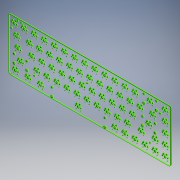
# Autodesk Inventor part: 60pc_pcb.kicad_v1.1_pcb.kicad_pcb
Saved by Autodesk Inventor 2018 (Build 220112000, 112)
## iProperties
Created: 2018-02-17
Part Number: 60pc_pcb.kicad_v1.1_pcb.kicad_pcb
Material: Generic
Document SubType Name: Modeling
Designer: ConnorDevitt
Density: 1 g/cm^3
Appearance: Board Outline
Author: ConnorDevitt
Autodesk Inventor part; units mm, degrees
(part 1 of 2)
ref_plane "YZ Plane" through (0, 0, 0) normal (1, 0, 0) x (0, 1, 0)
ref_plane "XZ Plane" through (0, 0, 0) normal (0, 1, 0) x (-1, 0, 0)
ref_plane "XY Plane" through (0, 0, 0) normal (0, 0, 1) x (1, 0, 0)
sketch "Sketch1" plane through (0, 0, 0) normal (0, 0, 1) x (1, 0, 0)
  line L0 (-153.375, 46.5) -> (-153.375, 43.75)
  line L1 (-153.375, 43.75) -> (-153.375, -45.25)
  arc A0 (-153.375, -45.25) -> (-149.375, -49.25) centre (-149.375, -45.25) ccw
  line L2 (-149.375, -49.25) -> (-147.625, -49.25)
  line L3 (-147.625, -49.25) -> (142.375, -49.25)
  line L4 (142.375, -49.25) -> (145.625, -49.25)
  line L5 (145.625, -49.25) -> (146.875, -49.25)
  line L6 (146.875, -49.25) -> (149.375, -49.25)
  arc A1 (149.375, -49.25) -> (153.375, -45.25) centre (149.375, -45.25) ccw
  line L7 (153.375, -45.25) -> (153.375, -18.5)
  line L8 (153.375, -18.5) -> (153.375, 46.5)
  arc A2 (153.375, 46.5) -> (150.625, 49.25) centre (150.625, 46.5) ccw
  line L9 (150.625, 49.25) -> (150.125, 49.25)
  line L10 (150.125, 49.25) -> (148.125, 49.25)
  line L11 (148.125, 49.25) -> (140.875, 49.25)
  line L12 (140.875, 49.25) -> (-127.875, 49.25)
  line L13 (-127.875, 49.25) -> (-128.125, 49.25)
  line L14 (-128.125, 49.25) -> (-148.875, 49.25)
  line L15 (-148.875, 49.25) -> (-150.625, 49.25)
  arc A3 (-150.625, 49.25) -> (-153.375, 46.5) centre (-150.625, 46.5) ccw
  line L16 (-126.3127, 41.7733) -> (-127.1236, 40.3134)
  arc A4 (-128.4349, 41.0417) -> (-127.1236, 40.3134) centre (-127.7792, 40.6775) ccw
  line L17 (-128.4349, 41.0417) -> (-127.6239, 42.5016)
  arc A5 (-126.3127, 41.7733) -> (-127.6239, 42.5016) centre (-126.9683, 42.1375) ccw
  line L18 (-120.6808, 43.1658) -> (-120.7202, 42.5872)
  arc A6 (-122.2167, 42.6892) -> (-120.7202, 42.5872) centre (-121.4685, 42.6382) ccw
  line L19 (-122.2167, 42.6892) -> (-122.1773, 43.2678)
  arc A7 (-120.6808, 43.1658) -> (-122.1773, 43.2678) centre (-121.429, 43.2168) ccw
  line L20 (-145.3627, 41.7733) -> (-146.1736, 40.3134)
  arc A8 (-147.4848, 41.0417) -> (-146.1736, 40.3134) centre (-146.8292, 40.6775) ccw
  line L21 (-147.4848, 41.0417) -> (-146.6739, 42.5016)
  arc A9 (-145.3627, 41.7733) -> (-146.6739, 42.5016) centre (-146.0183, 42.1375) ccw
  line L22 (-139.7308, 43.1658) -> (-139.7702, 42.5872)
  arc A10 (-141.2667, 42.6892) -> (-139.7702, 42.5872) centre (-140.5185, 42.6382) ccw
  line L23 (-141.2667, 42.6892) -> (-141.2273, 43.2678)
  arc A11 (-139.7308, 43.1658) -> (-141.2273, 43.2678) centre (-140.479, 43.2168) ccw
  line L24 (-136.925, 46.4) -> (-136.925, 43.9)
  arc A12 (-137.625, 43.9) -> (-136.925, 43.9) centre (-137.275, 43.9) ccw
  line L25 (-137.625, 43.9) -> (-137.625, 46.4)
  arc A13 (-136.925, 46.4) -> (-137.625, 46.4) centre (-137.275, 46.4) ccw
  line L26 (-129.625, 46.4) -> (-129.625, 43.9)
  arc A14 (-130.325, 43.9) -> (-129.625, 43.9) centre (-129.975, 43.9) ccw
  line L27 (-130.325, 43.9) -> (-130.325, 46.4)
  arc A15 (-129.625, 46.4) -> (-130.325, 46.4) centre (-129.975, 46.4) ccw
  line L28 (-140.6002, 22.7233) -> (-141.4111, 21.2634)
  arc A16 (-142.7224, 21.9917) -> (-141.4111, 21.2634) centre (-142.0667, 21.6275) ccw
  line L29 (-142.7224, 21.9917) -> (-141.9114, 23.4516)
  arc A17 (-140.6002, 22.7233) -> (-141.9114, 23.4516) centre (-141.2558, 23.0875) ccw
  line L30 (-134.9683, 24.1158) -> (-135.0077, 23.5372)
  arc A18 (-136.5042, 23.6392) -> (-135.0077, 23.5372) centre (-135.756, 23.5882) ccw
  line L31 (-136.5042, 23.6392) -> (-136.4648, 24.2178)
  arc A19 (-134.9683, 24.1158) -> (-136.4648, 24.2178) centre (-135.7165, 24.1668) ccw
  line L32 (-138.2189, 3.6733) -> (-139.0298, 2.2134)
  arc A20 (-140.3411, 2.9417) -> (-139.0298, 2.2134) centre (-139.6855, 2.5775) ccw
  line L33 (-140.3411, 2.9417) -> (-139.5302, 4.4016)
  arc A21 (-138.2189, 3.6733) -> (-139.5302, 4.4016) centre (-138.8745, 4.0375) ccw
  line L34 (-132.587, 5.0658) -> (-132.6265, 4.4872)
  arc A22 (-134.123, 4.5892) -> (-132.6265, 4.4872) centre (-133.3747, 4.5382) ccw
  line L35 (-134.123, 4.5892) -> (-134.0835, 5.1678)
  arc A23 (-132.587, 5.0658) -> (-134.0835, 5.1678) centre (-133.3353, 5.1168) ccw
  line L36 (-133.4564, -15.3767) -> (-134.2673, -16.8366)
  arc A24 (-135.5786, -16.1083) -> (-134.2673, -16.8366) centre (-134.923, -16.4725) ccw
  line L37 (-135.5786, -16.1083) -> (-134.7677, -14.6484)
  arc A25 (-133.4564, -15.3767) -> (-134.7677, -14.6484) centre (-134.112, -15.0125) ccw
  line L38 (-127.8245, -13.9842) -> (-127.864, -14.5628)
  arc A26 (-129.3605, -14.4608) -> (-127.864, -14.5628) centre (-128.6122, -14.5118) ccw
  line L39 (-129.3605, -14.4608) -> (-129.321, -13.8822)
  arc A27 (-127.8245, -13.9842) -> (-129.321, -13.8822) centre (-128.5728, -13.9332) ccw
  line L40 (-142.9814, -34.4267) -> (-143.7923, -35.8866)
  arc A28 (-145.1036, -35.1583) -> (-143.7923, -35.8866) centre (-144.448, -35.5225) ccw
  line L41 (-145.1036, -35.1583) -> (-144.2927, -33.6984)
  arc A29 (-142.9814, -34.4267) -> (-144.2927, -33.6984) centre (-143.637, -34.0625) ccw
  line L42 (-137.3495, -33.0342) -> (-137.389, -33.6128)
  arc A30 (-138.8855, -33.5108) -> (-137.389, -33.6128) centre (-138.1372, -33.5618) ccw
  line L43 (-138.8855, -33.5108) -> (-138.846, -32.9322)
  arc A31 (-137.3495, -33.0342) -> (-138.846, -32.9322) centre (-138.0978, -32.9832) ccw
  line L44 (-116.7876, 22.7233) -> (-117.5986, 21.2634)
  arc A32 (-118.9099, 21.9917) -> (-117.5986, 21.2634) centre (-118.2542, 21.6275) ccw
  line L45 (-118.9099, 21.9917) -> (-118.0989, 23.4516)
  arc A33 (-116.7876, 22.7233) -> (-118.0989, 23.4516) centre (-117.4433, 23.0875) ccw
  line L46 (-111.1558, 24.1158) -> (-111.1952, 23.5372)
  arc A34 (-112.6917, 23.6392) -> (-111.1952, 23.5372) centre (-111.9435, 23.5882) ccw
  line L47 (-112.6917, 23.6392) -> (-112.6523, 24.2178)
  arc A35 (-111.1558, 24.1158) -> (-112.6523, 24.2178) centre (-111.904, 24.1668) ccw
  line L48 (-112.0251, 3.6733) -> (-112.8361, 2.2134)
  arc A36 (-114.1474, 2.9417) -> (-112.8361, 2.2134) centre (-113.4917, 2.5775) ccw
  line L49 (-114.1474, 2.9417) -> (-113.3364, 4.4016)
  arc A37 (-112.0251, 3.6733) -> (-113.3364, 4.4016) centre (-112.6808, 4.0375) ccw
  line L50 (-106.3933, 5.0658) -> (-106.4327, 4.4872)
  arc A38 (-107.9292, 4.5892) -> (-106.4327, 4.4872) centre (-107.181, 4.5382) ccw
  line L51 (-107.9292, 4.5892) -> (-107.8898, 5.1678)
  arc A39 (-106.3933, 5.0658) -> (-107.8898, 5.1678) centre (-107.1415, 5.1168) ccw
  line L52 (-102.5002, -15.3767) -> (-103.3111, -16.8366)
  arc A40 (-104.6223, -16.1083) -> (-103.3111, -16.8366) centre (-103.9667, -16.4725) ccw
  line L53 (-104.6223, -16.1083) -> (-103.8114, -14.6484)
  arc A41 (-102.5002, -15.3767) -> (-103.8114, -14.6484) centre (-103.1558, -15.0125) ccw
  line L54 (-96.8683, -13.9842) -> (-96.9077, -14.5628)
  arc A42 (-98.4042, -14.4608) -> (-96.9077, -14.5628) centre (-97.656, -14.5118) ccw
  line L55 (-98.4042, -14.4608) -> (-98.3648, -13.8822)
  arc A43 (-96.8683, -13.9842) -> (-98.3648, -13.8822) centre (-97.6165, -13.9332) ccw
  line L56 (-119.1689, -34.4267) -> (-119.9798, -35.8866)
  arc A44 (-121.2911, -35.1583) -> (-119.9798, -35.8866) centre (-120.6355, -35.5225) ccw
  line L57 (-121.2911, -35.1583) -> (-120.4802, -33.6984)
  arc A45 (-119.1689, -34.4267) -> (-120.4802, -33.6984) centre (-119.8245, -34.0625) ccw
  line L58 (-113.537, -33.0342) -> (-113.5765, -33.6128)
  arc A46 (-115.073, -33.5108) -> (-113.5765, -33.6128) centre (-114.3247, -33.5618) ccw
  line L59 (-115.073, -33.5108) -> (-115.0335, -32.9322)
  arc A47 (-113.537, -33.0342) -> (-115.0335, -32.9322) centre (-114.2853, -32.9832) ccw
  line L60 (-95.3564, -34.4267) -> (-96.1673, -35.8866)
  arc A48 (-97.4786, -35.1583) -> (-96.1673, -35.8866) centre (-96.823, -35.5225) ccw
  line L61 (-97.4786, -35.1583) -> (-96.6677, -33.6984)
  arc A49 (-95.3564, -34.4267) -> (-96.6677, -33.6984) centre (-96.012, -34.0625) ccw
  line L62 (-89.7245, -33.0342) -> (-89.764, -33.6128)
  arc A50 (-91.2605, -33.5108) -> (-89.764, -33.6128) centre (-90.5122, -33.5618) ccw
  line L63 (-91.2605, -33.5108) -> (-91.221, -32.9322)
  arc A51 (-89.7245, -33.0342) -> (-91.221, -32.9322) centre (-90.4728, -32.9832) ccw
  line L64 (-107.2626, 41.7733) -> (-108.0736, 40.3134)
  arc A52 (-109.3849, 41.0417) -> (-108.0736, 40.3134) centre (-108.7292, 40.6775) ccw
  line L65 (-109.3849, 41.0417) -> (-108.5739, 42.5016)
  arc A53 (-107.2626, 41.7733) -> (-108.5739, 42.5016) centre (-107.9183, 42.1375) ccw
  line L66 (-101.6308, 43.1658) -> (-101.6702, 42.5872)
  arc A54 (-103.1667, 42.6892) -> (-101.6702, 42.5872) centre (-102.4185, 42.6382) ccw
  line L67 (-103.1667, 42.6892) -> (-103.1273, 43.2678)
  arc A55 (-101.6308, 43.1658) -> (-103.1273, 43.2678) centre (-102.379, 43.2168) ccw
  line L68 (-97.7377, 22.7233) -> (-98.5486, 21.2634)
  arc A56 (-99.8598, 21.9917) -> (-98.5486, 21.2634) centre (-99.2042, 21.6275) ccw
  line L69 (-99.8598, 21.9917) -> (-99.0489, 23.4516)
  arc A57 (-97.7377, 22.7233) -> (-99.0489, 23.4516) centre (-98.3933, 23.0875) ccw
  line L70 (-92.1058, 24.1158) -> (-92.1452, 23.5372)
  arc A58 (-93.6417, 23.6392) -> (-92.1452, 23.5372) centre (-92.8935, 23.5882) ccw
  line L71 (-93.6417, 23.6392) -> (-93.6023, 24.2178)
  arc A59 (-92.1058, 24.1158) -> (-93.6023, 24.2178) centre (-92.854, 24.1668) ccw
  line L72 (-92.9752, 3.6733) -> (-93.7861, 2.2134)
  arc A60 (-95.0974, 2.9417) -> (-93.7861, 2.2134) centre (-94.4417, 2.5775) ccw
  line L73 (-95.0974, 2.9417) -> (-94.2864, 4.4016)
  arc A61 (-92.9752, 3.6733) -> (-94.2864, 4.4016) centre (-93.6308, 4.0375) ccw
  line L74 (-87.3433, 5.0658) -> (-87.3827, 4.4872)
  arc A62 (-88.8792, 4.5892) -> (-87.3827, 4.4872) centre (-88.131, 4.5382) ccw
  line L75 (-88.8792, 4.5892) -> (-88.8398, 5.1678)
  arc A63 (-87.3433, 5.0658) -> (-88.8398, 5.1678) centre (-88.0915, 5.1168) ccw
  line L76 (-83.4502, -15.3767) -> (-84.2611, -16.8366)
  arc A64 (-85.5724, -16.1083) -> (-84.2611, -16.8366) centre (-84.9167, -16.4725) ccw
  line L77 (-85.5724, -16.1083) -> (-84.7614, -14.6484)
  arc A65 (-83.4502, -15.3767) -> (-84.7614, -14.6484) centre (-84.1058, -15.0125) ccw
  line L78 (-77.8183, -13.9842) -> (-77.8577, -14.5628)
  arc A66 (-79.3542, -14.4608) -> (-77.8577, -14.5628) centre (-78.606, -14.5118) ccw
  line L79 (-79.3542, -14.4608) -> (-79.3148, -13.8822)
  arc A67 (-77.8183, -13.9842) -> (-79.3148, -13.8822) centre (-78.5665, -13.9332) ccw
  line L80 (-88.2126, 41.7733) -> (-89.0236, 40.3134)
  arc A68 (-90.3349, 41.0417) -> (-89.0236, 40.3134) centre (-89.6792, 40.6775) ccw
  line L81 (-90.3349, 41.0417) -> (-89.5239, 42.5016)
  arc A69 (-88.2126, 41.7733) -> (-89.5239, 42.5016) centre (-88.8683, 42.1375) ccw
  line L82 (-82.5808, 43.1658) -> (-82.6202, 42.5872)
  arc A70 (-84.1167, 42.6892) -> (-82.6202, 42.5872) centre (-83.3685, 42.6382) ccw
  line L83 (-84.1167, 42.6892) -> (-84.0773, 43.2678)
  arc A71 (-82.5808, 43.1658) -> (-84.0773, 43.2678) centre (-83.329, 43.2168) ccw
  line L84 (-78.6877, 22.7233) -> (-79.4986, 21.2634)
  arc A72 (-80.8098, 21.9917) -> (-79.4986, 21.2634) centre (-80.1542, 21.6275) ccw
  line L85 (-80.8098, 21.9917) -> (-79.9989, 23.4516)
  arc A73 (-78.6877, 22.7233) -> (-79.9989, 23.4516) centre (-79.3433, 23.0875) ccw
  line L86 (-73.0558, 24.1158) -> (-73.0952, 23.5372)
  arc A74 (-74.5917, 23.6392) -> (-73.0952, 23.5372) centre (-73.8435, 23.5882) ccw
  line L87 (-74.5917, 23.6392) -> (-74.5523, 24.2178)
  arc A75 (-73.0558, 24.1158) -> (-74.5523, 24.2178) centre (-73.804, 24.1668) ccw
  line L88 (-73.9252, 3.6733) -> (-74.7361, 2.2134)
  arc A76 (-76.0473, 2.9417) -> (-74.7361, 2.2134) centre (-75.3917, 2.5775) ccw
  line L89 (-76.0473, 2.9417) -> (-75.2364, 4.4016)
  arc A77 (-73.9252, 3.6733) -> (-75.2364, 4.4016) centre (-74.5808, 4.0375) ccw
  line L90 (-68.2933, 5.0658) -> (-68.3327, 4.4872)
  arc A78 (-69.8292, 4.5892) -> (-68.3327, 4.4872) centre (-69.081, 4.5382) ccw
  line L91 (-69.8292, 4.5892) -> (-69.7898, 5.1678)
  arc A79 (-68.2933, 5.0658) -> (-69.7898, 5.1678) centre (-69.0415, 5.1168) ccw
  line L92 (-64.4001, -15.3767) -> (-65.2111, -16.8366)
  arc A80 (-66.5224, -16.1083) -> (-65.2111, -16.8366) centre (-65.8667, -16.4725) ccw
  line L93 (-66.5224, -16.1083) -> (-65.7114, -14.6484)
  arc A81 (-64.4001, -15.3767) -> (-65.7114, -14.6484) centre (-65.0558, -15.0125) ccw
  line L94 (-58.7683, -13.9842) -> (-58.8077, -14.5628)
  arc A82 (-60.3042, -14.4608) -> (-58.8077, -14.5628) centre (-59.556, -14.5118) ccw
  line L95 (-60.3042, -14.4608) -> (-60.2648, -13.8822)
  arc A83 (-58.7683, -13.9842) -> (-60.2648, -13.8822) centre (-59.5165, -13.9332) ccw
  line L96 (-69.1626, 41.7733) -> (-69.9736, 40.3134)
  arc A84 (-71.2849, 41.0417) -> (-69.9736, 40.3134) centre (-70.6292, 40.6775) ccw
  line L97 (-71.2849, 41.0417) -> (-70.4739, 42.5016)
  arc A85 (-69.1626, 41.7733) -> (-70.4739, 42.5016) centre (-69.8183, 42.1375) ccw
  line L98 (-63.5308, 43.1658) -> (-63.5702, 42.5872)
  arc A86 (-65.0667, 42.6892) -> (-63.5702, 42.5872) centre (-64.3185, 42.6382) ccw
  line L99 (-65.0667, 42.6892) -> (-65.0273, 43.2678)
  arc A87 (-63.5308, 43.1658) -> (-65.0273, 43.2678) centre (-64.279, 43.2168) ccw
  line L100 (-59.6377, 22.7233) -> (-60.4486, 21.2634)
  arc A88 (-61.7599, 21.9917) -> (-60.4486, 21.2634) centre (-61.1042, 21.6275) ccw
  line L101 (-61.7599, 21.9917) -> (-60.9489, 23.4516)
  arc A89 (-59.6377, 22.7233) -> (-60.9489, 23.4516) centre (-60.2933, 23.0875) ccw
  line L102 (-54.0058, 24.1158) -> (-54.0452, 23.5372)
  arc A90 (-55.5417, 23.6392) -> (-54.0452, 23.5372) centre (-54.7935, 23.5882) ccw
  line L103 (-55.5417, 23.6392) -> (-55.5023, 24.2178)
  arc A91 (-54.0058, 24.1158) -> (-55.5023, 24.2178) centre (-54.754, 24.1668) ccw
  line L104 (-54.8752, 3.6733) -> (-55.6861, 2.2134)
  arc A92 (-56.9974, 2.9417) -> (-55.6861, 2.2134) centre (-56.3417, 2.5775) ccw
  line L105 (-56.9974, 2.9417) -> (-56.1864, 4.4016)
  arc A93 (-54.8752, 3.6733) -> (-56.1864, 4.4016) centre (-55.5308, 4.0375) ccw
  line L106 (-49.2433, 5.0658) -> (-49.2827, 4.4872)
  arc A94 (-50.7792, 4.5892) -> (-49.2827, 4.4872) centre (-50.031, 4.5382) ccw
  line L107 (-50.7792, 4.5892) -> (-50.7398, 5.1678)
  arc A95 (-49.2433, 5.0658) -> (-50.7398, 5.1678) centre (-49.9915, 5.1168) ccw
  line L108 (-45.3502, -15.3767) -> (-46.1611, -16.8366)
  arc A96 (-47.4723, -16.1083) -> (-46.1611, -16.8366) centre (-46.8167, -16.4725) ccw
  line L109 (-47.4723, -16.1083) -> (-46.6614, -14.6484)
  arc A97 (-45.3502, -15.3767) -> (-46.6614, -14.6484) centre (-46.0058, -15.0125) ccw
  line L110 (-39.7183, -13.9842) -> (-39.7577, -14.5628)
  arc A98 (-41.2542, -14.4608) -> (-39.7577, -14.5628) centre (-40.506, -14.5118) ccw
  line L111 (-41.2542, -14.4608) -> (-41.2148, -13.8822)
  arc A99 (-39.7183, -13.9842) -> (-41.2148, -13.8822) centre (-40.4665, -13.9332) ccw
  line L112 (-50.1127, 41.7733) -> (-50.9236, 40.3134)
  arc A100 (-52.2349, 41.0417) -> (-50.9236, 40.3134) centre (-51.5792, 40.6775) ccw
  line L113 (-52.2349, 41.0417) -> (-51.4239, 42.5016)
  arc A101 (-50.1127, 41.7733) -> (-51.4239, 42.5016) centre (-50.7683, 42.1375) ccw
  line L114 (-44.4808, 43.1658) -> (-44.5202, 42.5872)
  arc A102 (-46.0167, 42.6892) -> (-44.5202, 42.5872) centre (-45.2685, 42.6382) ccw
  line L115 (-46.0167, 42.6892) -> (-45.9773, 43.2678)
  arc A103 (-44.4808, 43.1658) -> (-45.9773, 43.2678) centre (-45.229, 43.2168) ccw
  line L116 (-40.5877, 22.7233) -> (-41.3986, 21.2634)
  arc A104 (-42.7099, 21.9917) -> (-41.3986, 21.2634) centre (-42.0542, 21.6275) ccw
  line L117 (-42.7099, 21.9917) -> (-41.8989, 23.4516)
  arc A105 (-40.5877, 22.7233) -> (-41.8989, 23.4516) centre (-41.2433, 23.0875) ccw
  line L118 (-34.9558, 24.1158) -> (-34.9952, 23.5372)
  arc A106 (-36.4917, 23.6392) -> (-34.9952, 23.5372) centre (-35.7435, 23.5882) ccw
  line L119 (-36.4917, 23.6392) -> (-36.4523, 24.2178)
  arc A107 (-34.9558, 24.1158) -> (-36.4523, 24.2178) centre (-35.704, 24.1668) ccw
  line L120 (-35.8252, 3.6733) -> (-36.6361, 2.2134)
  arc A108 (-37.9474, 2.9417) -> (-36.6361, 2.2134) centre (-37.2917, 2.5775) ccw
  line L121 (-37.9474, 2.9417) -> (-37.1364, 4.4016)
  arc A109 (-35.8252, 3.6733) -> (-37.1364, 4.4016) centre (-36.4808, 4.0375) ccw
  line L122 (-30.1933, 5.0658) -> (-30.2327, 4.4872)
  arc A110 (-31.7292, 4.5892) -> (-30.2327, 4.4872) centre (-30.981, 4.5382) ccw
  line L123 (-31.7292, 4.5892) -> (-31.6898, 5.1678)
  arc A111 (-30.1933, 5.0658) -> (-31.6898, 5.1678) centre (-30.9415, 5.1168) ccw
  line L124 (-26.3002, -15.3767) -> (-27.1111, -16.8366)
  arc A112 (-28.4224, -16.1083) -> (-27.1111, -16.8366) centre (-27.7667, -16.4725) ccw
  line L125 (-28.4224, -16.1083) -> (-27.6114, -14.6484)
  arc A113 (-26.3002, -15.3767) -> (-27.6114, -14.6484) centre (-26.9558, -15.0125) ccw
  line L126 (-20.6683, -13.9842) -> (-20.7077, -14.5628)
  arc A114 (-22.2042, -14.4608) -> (-20.7077, -14.5628) centre (-21.456, -14.5118) ccw
  line L127 (-22.2042, -14.4608) -> (-22.1648, -13.8822)
  arc A115 (-20.6683, -13.9842) -> (-22.1648, -13.8822) centre (-21.4165, -13.9332) ccw
  line L128 (-31.0627, 41.7733) -> (-31.8736, 40.3134)
  arc A116 (-33.1848, 41.0417) -> (-31.8736, 40.3134) centre (-32.5292, 40.6775) ccw
  line L129 (-33.1848, 41.0417) -> (-32.3739, 42.5016)
  arc A117 (-31.0627, 41.7733) -> (-32.3739, 42.5016) centre (-31.7183, 42.1375) ccw
  line L130 (-25.4308, 43.1658) -> (-25.4702, 42.5872)
  arc A118 (-26.9667, 42.6892) -> (-25.4702, 42.5872) centre (-26.2185, 42.6382) ccw
  line L131 (-26.9667, 42.6892) -> (-26.9273, 43.2678)
  arc A119 (-25.4308, 43.1658) -> (-26.9273, 43.2678) centre (-26.179, 43.2168) ccw
  line L132 (-21.5376, 22.7233) -> (-22.3486, 21.2634)
  arc A120 (-23.6598, 21.9917) -> (-22.3486, 21.2634) centre (-23.0042, 21.6275) ccw
  line L133 (-23.6598, 21.9917) -> (-22.8489, 23.4516)
  arc A121 (-21.5376, 22.7233) -> (-22.8489, 23.4516) centre (-22.1933, 23.0875) ccw
  line L134 (-15.9058, 24.1158) -> (-15.9452, 23.5372)
  arc A122 (-17.4417, 23.6392) -> (-15.9452, 23.5372) centre (-16.6935, 23.5882) ccw
  line L135 (-17.4417, 23.6392) -> (-17.4023, 24.2178)
  arc A123 (-15.9058, 24.1158) -> (-17.4023, 24.2178) centre (-16.654, 24.1668) ccw
  line L136 (-16.7752, 3.6733) -> (-17.5861, 2.2134)
  arc A124 (-18.8973, 2.9417) -> (-17.5861, 2.2134) centre (-18.2417, 2.5775) ccw
  line L137 (-18.8973, 2.9417) -> (-18.0864, 4.4016)
  arc A125 (-16.7752, 3.6733) -> (-18.0864, 4.4016) centre (-17.4308, 4.0375) ccw
  line L138 (-11.1433, 5.0658) -> (-11.1827, 4.4872)
  arc A126 (-12.6792, 4.5892) -> (-11.1827, 4.4872) centre (-11.931, 4.5382) ccw
  line L139 (-12.6792, 4.5892) -> (-12.6398, 5.1678)
  arc A127 (-11.1433, 5.0658) -> (-12.6398, 5.1678) centre (-11.8915, 5.1168) ccw
  line L140 (-7.2501, -15.3767) -> (-8.0611, -16.8366)
  arc A128 (-9.3724, -16.1083) -> (-8.0611, -16.8366) centre (-8.7167, -16.4725) ccw
  line L141 (-9.3724, -16.1083) -> (-8.5614, -14.6484)
  arc A129 (-7.2501, -15.3767) -> (-8.5614, -14.6484) centre (-7.9058, -15.0125) ccw
  line L142 (-1.6183, -13.9842) -> (-1.6577, -14.5628)
  arc A130 (-3.1542, -14.4608) -> (-1.6577, -14.5628) centre (-2.406, -14.5118) ccw
  line L143 (-3.1542, -14.4608) -> (-3.1148, -13.8822)
  arc A131 (-1.6183, -13.9842) -> (-3.1148, -13.8822) centre (-2.3665, -13.9332) ccw
  line L144 (-23.9189, -34.4267) -> (-24.7298, -35.8866)
  arc A132 (-26.0411, -35.1583) -> (-24.7298, -35.8866) centre (-25.3855, -35.5225) ccw
  line L145 (-26.0411, -35.1583) -> (-25.2302, -33.6984)
  arc A133 (-23.9189, -34.4267) -> (-25.2302, -33.6984) centre (-24.5745, -34.0625) ccw
  line L146 (-18.287, -33.0342) -> (-18.3265, -33.6128)
  arc A134 (-19.823, -33.5108) -> (-18.3265, -33.6128) centre (-19.0747, -33.5618) ccw
  line L147 (-19.823, -33.5108) -> (-19.7835, -32.9322)
  arc A135 (-18.287, -33.0342) -> (-19.7835, -32.9322) centre (-19.0353, -32.9832) ccw
  line L148 (-12.0127, 41.7733) -> (-12.8236, 40.3134)
  arc A136 (-14.1349, 41.0417) -> (-12.8236, 40.3134) centre (-13.4792, 40.6775) ccw
  line L149 (-14.1349, 41.0417) -> (-13.3239, 42.5016)
  arc A137 (-12.0127, 41.7733) -> (-13.3239, 42.5016) centre (-12.6683, 42.1375) ccw
  line L150 (-6.3808, 43.1658) -> (-6.4202, 42.5872)
  arc A138 (-7.9167, 42.6892) -> (-6.4202, 42.5872) centre (-7.1685, 42.6382) ccw
  line L151 (-7.9167, 42.6892) -> (-7.8773, 43.2678)
  arc A139 (-6.3808, 43.1658) -> (-7.8773, 43.2678) centre (-7.129, 43.2168) ccw
  line L152 (-2.4877, 22.7233) -> (-3.2986, 21.2634)
  arc A140 (-4.6098, 21.9917) -> (-3.2986, 21.2634) centre (-3.9542, 21.6275) ccw
  line L153 (-4.6098, 21.9917) -> (-3.7989, 23.4516)
  arc A141 (-2.4877, 22.7233) -> (-3.7989, 23.4516) centre (-3.1433, 23.0875) ccw
  line L154 (3.1442, 24.1158) -> (3.1048, 23.5372)
  arc A142 (1.6083, 23.6392) -> (3.1048, 23.5372) centre (2.3565, 23.5882) ccw
  line L155 (1.6083, 23.6392) -> (1.6477, 24.2178)
  arc A143 (3.1442, 24.1158) -> (1.6477, 24.2178) centre (2.396, 24.1668) ccw
  line L156 (2.2748, 3.6733) -> (1.4639, 2.2134)
  arc A144 (0.1527, 2.9417) -> (1.4639, 2.2134) centre (0.8083, 2.5775) ccw
  line L157 (0.1527, 2.9417) -> (0.9636, 4.4016)
  arc A145 (2.2748, 3.6733) -> (0.9636, 4.4016) centre (1.6192, 4.0375) ccw
  line L158 (7.9067, 5.0658) -> (7.8673, 4.4872)
  arc A146 (6.3708, 4.5892) -> (7.8673, 4.4872) centre (7.119, 4.5382) ccw
  line L159 (6.3708, 4.5892) -> (6.4102, 5.1678)
  arc A147 (7.9067, 5.0658) -> (6.4102, 5.1678) centre (7.1585, 5.1168) ccw
  line L160 (11.7999, -15.3767) -> (10.9889, -16.8366)
  arc A148 (9.6776, -16.1083) -> (10.9889, -16.8366) centre (10.3333, -16.4725) ccw
  line L161 (9.6776, -16.1083) -> (10.4886, -14.6484)
  arc A149 (11.7999, -15.3767) -> (10.4886, -14.6484) centre (11.1442, -15.0125) ccw
  line L162 (17.4317, -13.9842) -> (17.3923, -14.5628)
  arc A150 (15.8958, -14.4608) -> (17.3923, -14.5628) centre (16.644, -14.5118) ccw
  line L163 (15.8958, -14.4608) -> (15.9352, -13.8822)
  arc A151 (17.4317, -13.9842) -> (15.9352, -13.8822) centre (16.6835, -13.9332) ccw
  line L164 (7.0373, 41.7733) -> (6.2264, 40.3134)
  arc A152 (4.9151, 41.0417) -> (6.2264, 40.3134) centre (5.5708, 40.6775) ccw
  line L165 (4.9151, 41.0417) -> (5.7261, 42.5016)
  arc A153 (7.0373, 41.7733) -> (5.7261, 42.5016) centre (6.3817, 42.1375) ccw
  line L166 (12.6692, 43.1658) -> (12.6298, 42.5872)
  arc A154 (11.1333, 42.6892) -> (12.6298, 42.5872) centre (11.8815, 42.6382) ccw
  line L167 (11.1333, 42.6892) -> (11.1727, 43.2678)
  arc A155 (12.6692, 43.1658) -> (11.1727, 43.2678) centre (11.921, 43.2168) ccw
  line L168 (16.5623, 22.7233) -> (15.7514, 21.2634)
  arc A156 (14.4402, 21.9917) -> (15.7514, 21.2634) centre (15.0958, 21.6275) ccw
  line L169 (14.4402, 21.9917) -> (15.2511, 23.4516)
  arc A157 (16.5623, 22.7233) -> (15.2511, 23.4516) centre (15.9067, 23.0875) ccw
  line L170 (22.1942, 24.1158) -> (22.1548, 23.5372)
  arc A158 (20.6583, 23.6392) -> (22.1548, 23.5372) centre (21.4065, 23.5882) ccw
  line L171 (20.6583, 23.6392) -> (20.6977, 24.2178)
  arc A159 (22.1942, 24.1158) -> (20.6977, 24.2178) centre (21.446, 24.1668) ccw
  line L172 (21.3249, 3.6733) -> (20.5139, 2.2134)
  arc A160 (19.2026, 2.9417) -> (20.5139, 2.2134) centre (19.8583, 2.5775) ccw
  line L173 (19.2026, 2.9417) -> (20.0136, 4.4016)
  arc A161 (21.3249, 3.6733) -> (20.0136, 4.4016) centre (20.6692, 4.0375) ccw
  line L174 (26.9567, 5.0658) -> (26.9173, 4.4872)
  arc A162 (25.4208, 4.5892) -> (26.9173, 4.4872) centre (26.169, 4.5382) ccw
  line L175 (25.4208, 4.5892) -> (25.4602, 5.1678)
  arc A163 (26.9567, 5.0658) -> (25.4602, 5.1678) centre (26.2085, 5.1168) ccw
  line L176 (30.8498, -15.3767) -> (30.0389, -16.8366)
  arc A164 (28.7277, -16.1083) -> (30.0389, -16.8366) centre (29.3833, -16.4725) ccw
  line L177 (28.7277, -16.1083) -> (29.5386, -14.6484)
  arc A165 (30.8498, -15.3767) -> (29.5386, -14.6484) centre (30.1942, -15.0125) ccw
  line L178 (36.4817, -13.9842) -> (36.4423, -14.5628)
  arc A166 (34.9458, -14.4608) -> (36.4423, -14.5628) centre (35.694, -14.5118) ccw
  line L179 (34.9458, -14.4608) -> (34.9852, -13.8822)
  arc A167 (36.4817, -13.9842) -> (34.9852, -13.8822) centre (35.7335, -13.9332) ccw
  line L180 (26.0874, 41.7733) -> (25.2764, 40.3134)
  arc A168 (23.9652, 41.0417) -> (25.2764, 40.3134) centre (24.6208, 40.6775) ccw
  line L181 (23.9652, 41.0417) -> (24.7761, 42.5016)
  arc A169 (26.0874, 41.7733) -> (24.7761, 42.5016) centre (25.4317, 42.1375) ccw
  line L182 (31.7192, 43.1658) -> (31.6798, 42.5872)
  arc A170 (30.1833, 42.6892) -> (31.6798, 42.5872) centre (30.9315, 42.6382) ccw
  line L183 (30.1833, 42.6892) -> (30.2227, 43.2678)
  arc A171 (31.7192, 43.1658) -> (30.2227, 43.2678) centre (30.971, 43.2168) ccw
  line L184 (35.6123, 22.7233) -> (34.8014, 21.2634)
  arc A172 (33.4901, 21.9917) -> (34.8014, 21.2634) centre (34.1458, 21.6275) ccw
  line L185 (33.4901, 21.9917) -> (34.3011, 23.4516)
  arc A173 (35.6123, 22.7233) -> (34.3011, 23.4516) centre (34.9567, 23.0875) ccw
  line L186 (41.2442, 24.1158) -> (41.2048, 23.5372)
  arc A174 (39.7083, 23.6392) -> (41.2048, 23.5372) centre (40.4565, 23.5882) ccw
  line L187 (39.7083, 23.6392) -> (39.7477, 24.2178)
  arc A175 (41.2442, 24.1158) -> (39.7477, 24.2178) centre (40.496, 24.1668) ccw
  line L188 (40.3749, 3.6733) -> (39.5639, 2.2134)
  arc A176 (38.2527, 2.9417) -> (39.5639, 2.2134) centre (38.9083, 2.5775) ccw
  line L189 (38.2527, 2.9417) -> (39.0636, 4.4016)
  arc A177 (40.3749, 3.6733) -> (39.0636, 4.4016) centre (39.7192, 4.0375) ccw
  line L190 (46.0067, 5.0658) -> (45.9673, 4.4872)
  arc A178 (44.4708, 4.5892) -> (45.9673, 4.4872) centre (45.219, 4.5382) ccw
  line L191 (44.4708, 4.5892) -> (44.5102, 5.1678)
  arc A179 (46.0067, 5.0658) -> (44.5102, 5.1678) centre (45.2585, 5.1168) ccw
  line L192 (49.8999, -15.3767) -> (49.0889, -16.8366)
  arc A180 (47.7777, -16.1083) -> (49.0889, -16.8366) centre (48.4333, -16.4725) ccw
  line L193 (47.7777, -16.1083) -> (48.5886, -14.6484)
  arc A181 (49.8999, -15.3767) -> (48.5886, -14.6484) centre (49.2442, -15.0125) ccw
  line L194 (55.5317, -13.9842) -> (55.4923, -14.5628)
  arc A182 (53.9958, -14.4608) -> (55.4923, -14.5628) centre (54.744, -14.5118) ccw
  line L195 (53.9958, -14.4608) -> (54.0352, -13.8822)
  arc A183 (55.5317, -13.9842) -> (54.0352, -13.8822) centre (54.7835, -13.9332) ccw
  line L196 (45.1373, 41.7733) -> (44.3264, 40.3134)
  arc A184 (43.0152, 41.0417) -> (44.3264, 40.3134) centre (43.6708, 40.6775) ccw
  line L197 (43.0152, 41.0417) -> (43.8261, 42.5016)
  arc A185 (45.1373, 41.7733) -> (43.8261, 42.5016) centre (44.4817, 42.1375) ccw
  line L198 (50.7692, 43.1658) -> (50.7298, 42.5872)
  arc A186 (49.2333, 42.6892) -> (50.7298, 42.5872) centre (49.9815, 42.6382) ccw
  line L199 (49.2333, 42.6892) -> (49.2727, 43.2678)
  arc A187 (50.7692, 43.1658) -> (49.2727, 43.2678) centre (50.021, 43.2168) ccw
  line L200 (54.6624, 22.7233) -> (53.8514, 21.2634)
  arc A188 (52.5401, 21.9917) -> (53.8514, 21.2634) centre (53.1958, 21.6275) ccw
  line L201 (52.5401, 21.9917) -> (53.3511, 23.4516)
  arc A189 (54.6624, 22.7233) -> (53.3511, 23.4516) centre (54.0067, 23.0875) ccw
  line L202 (60.2942, 24.1158) -> (60.2548, 23.5372)
  arc A190 (58.7583, 23.6392) -> (60.2548, 23.5372) centre (59.5065, 23.5882) ccw
  line L203 (58.7583, 23.6392) -> (58.7977, 24.2178)
  arc A191 (60.2942, 24.1158) -> (58.7977, 24.2178) centre (59.546, 24.1668) ccw
  line L204 (59.4249, 3.6733) -> (58.6139, 2.2134)
  arc A192 (57.3026, 2.9417) -> (58.6139, 2.2134) centre (57.9583, 2.5775) ccw
  line L205 (57.3026, 2.9417) -> (58.1136, 4.4016)
  arc A193 (59.4249, 3.6733) -> (58.1136, 4.4016) centre (58.7692, 4.0375) ccw
  line L206 (65.0567, 5.0658) -> (65.0173, 4.4872)
  arc A194 (63.5208, 4.5892) -> (65.0173, 4.4872) centre (64.269, 4.5382) ccw
  line L207 (63.5208, 4.5892) -> (63.5602, 5.1678)
  arc A195 (65.0567, 5.0658) -> (63.5602, 5.1678) centre (64.3085, 5.1168) ccw
  line L208 (68.9498, -15.3767) -> (68.1389, -16.8366)
  arc A196 (66.8277, -16.1083) -> (68.1389, -16.8366) centre (67.4833, -16.4725) ccw
  line L209 (66.8277, -16.1083) -> (67.6386, -14.6484)
  arc A197 (68.9498, -15.3767) -> (67.6386, -14.6484) centre (68.2942, -15.0125) ccw
  line L210 (74.5817, -13.9842) -> (74.5423, -14.5628)
  arc A198 (73.0458, -14.4608) -> (74.5423, -14.5628) centre (73.794, -14.5118) ccw
  line L211 (73.0458, -14.4608) -> (73.0852, -13.8822)
  arc A199 (74.5817, -13.9842) -> (73.0852, -13.8822) centre (73.8335, -13.9332) ccw
  line L212 (45.1373, -34.4267) -> (44.3264, -35.8866)
  arc A200 (43.0152, -35.1583) -> (44.3264, -35.8866) centre (43.6708, -35.5225) ccw
  line L213 (43.0152, -35.1583) -> (43.8261, -33.6984)
  arc A201 (45.1373, -34.4267) -> (43.8261, -33.6984) centre (44.4817, -34.0625) ccw
  line L214 (50.7692, -33.0342) -> (50.7298, -33.6128)
  arc A202 (49.2333, -33.5108) -> (50.7298, -33.6128) centre (49.9815, -33.5618) ccw
  line L215 (49.2333, -33.5108) -> (49.2727, -32.9322)
  arc A203 (50.7692, -33.0342) -> (49.2727, -32.9322) centre (50.021, -32.9832) ccw
  line L216 (64.1873, 41.7733) -> (63.3764, 40.3134)
  arc A204 (62.0652, 41.0417) -> (63.3764, 40.3134) centre (62.7208, 40.6775) ccw
  line L217 (62.0652, 41.0417) -> (62.8761, 42.5016)
  arc A205 (64.1873, 41.7733) -> (62.8761, 42.5016) centre (63.5317, 42.1375) ccw
  line L218 (69.8192, 43.1658) -> (69.7798, 42.5872)
  arc A206 (68.2833, 42.6892) -> (69.7798, 42.5872) centre (69.0315, 42.6382) ccw
  line L219 (68.2833, 42.6892) -> (68.3227, 43.2678)
  arc A207 (69.8192, 43.1658) -> (68.3227, 43.2678) centre (69.071, 43.2168) ccw
  line L220 (73.7124, 22.7233) -> (72.9014, 21.2634)
  arc A208 (71.5901, 21.9917) -> (72.9014, 21.2634) centre (72.2458, 21.6275) ccw
  line L221 (71.5901, 21.9917) -> (72.4011, 23.4516)
  arc A209 (73.7124, 22.7233) -> (72.4011, 23.4516) centre (73.0567, 23.0875) ccw
  line L222 (79.3442, 24.1158) -> (79.3048, 23.5372)
  arc A210 (77.8083, 23.6392) -> (79.3048, 23.5372) centre (78.5565, 23.5882) ccw
  line L223 (77.8083, 23.6392) -> (77.8477, 24.2178)
  arc A211 (79.3442, 24.1158) -> (77.8477, 24.2178) centre (78.596, 24.1668) ccw
  line L224 (78.4749, 3.6733) -> (77.6639, 2.2134)
  arc A212 (76.3527, 2.9417) -> (77.6639, 2.2134) centre (77.0083, 2.5775) ccw
  line L225 (76.3527, 2.9417) -> (77.1636, 4.4016)
  arc A213 (78.4749, 3.6733) -> (77.1636, 4.4016) centre (77.8192, 4.0375) ccw
  line L226 (84.1067, 5.0658) -> (84.0673, 4.4872)
  arc A214 (82.5708, 4.5892) -> (84.0673, 4.4872) centre (83.319, 4.5382) ccw
  line L227 (82.5708, 4.5892) -> (82.6102, 5.1678)
  arc A215 (84.1067, 5.0658) -> (82.6102, 5.1678) centre (83.3585, 5.1168) ccw
  line L228 (64.1873, -34.4267) -> (63.3764, -35.8866)
  arc A216 (62.0652, -35.1583) -> (63.3764, -35.8866) centre (62.7208, -35.5225) ccw
  line L229 (62.0652, -35.1583) -> (62.8761, -33.6984)
  arc A217 (64.1873, -34.4267) -> (62.8761, -33.6984) centre (63.5317, -34.0625) ccw
  line L230 (69.8192, -33.0342) -> (69.7798, -33.6128)
  arc A218 (68.2833, -33.5108) -> (69.7798, -33.6128) centre (69.0315, -33.5618) ccw
  line L231 (68.2833, -33.5108) -> (68.3227, -32.9322)
  arc A219 (69.8192, -33.0342) -> (68.3227, -32.9322) centre (69.071, -32.9832) ccw
  line L232 (83.2374, 41.7733) -> (82.4264, 40.3134)
  arc A220 (81.1151, 41.0417) -> (82.4264, 40.3134) centre (81.7708, 40.6775) ccw
  line L233 (81.1151, 41.0417) -> (81.9261, 42.5016)
  arc A221 (83.2374, 41.7733) -> (81.9261, 42.5016) centre (82.5817, 42.1375) ccw
  line L234 (88.8692, 43.1658) -> (88.8298, 42.5872)
  arc A222 (87.3333, 42.6892) -> (88.8298, 42.5872) centre (88.0815, 42.6382) ccw
  line L235 (87.3333, 42.6892) -> (87.3727, 43.2678)
  arc A223 (88.8692, 43.1658) -> (87.3727, 43.2678) centre (88.121, 43.2168) ccw
  line L236 (92.7623, 22.7233) -> (91.9514, 21.2634)
  arc A224 (90.6402, 21.9917) -> (91.9514, 21.2634) centre (91.2958, 21.6275) ccw
  line L237 (90.6402, 21.9917) -> (91.4511, 23.4516)
  arc A225 (92.7623, 22.7233) -> (91.4511, 23.4516) centre (92.1067, 23.0875) ccw
  line L238 (98.3942, 24.1158) -> (98.3548, 23.5372)
  arc A226 (96.8583, 23.6392) -> (98.3548, 23.5372) centre (97.6065, 23.5882) ccw
  line L239 (96.8583, 23.6392) -> (96.8977, 24.2178)
  arc A227 (98.3942, 24.1158) -> (96.8977, 24.2178) centre (97.646, 24.1668) ccw
  line L240 (109.4311, 3.6733) -> (108.6202, 2.2134)
  arc A228 (107.3089, 2.9417) -> (108.6202, 2.2134) centre (107.9645, 2.5775) ccw
  line L241 (107.3089, 2.9417) -> (108.1198, 4.4016)
  arc A229 (109.4311, 3.6733) -> (108.1198, 4.4016) centre (108.7755, 4.0375) ccw
  line L242 (115.063, 5.0658) -> (115.0235, 4.4872)
  arc A230 (113.527, 4.5892) -> (115.0235, 4.4872) centre (114.2753, 4.5382) ccw
  line L243 (113.527, 4.5892) -> (113.5665, 5.1678)
  arc A231 (115.063, 5.0658) -> (113.5665, 5.1678) centre (114.3147, 5.1168) ccw
  line L244 (121.3374, -15.3767) -> (120.5264, -16.8366)
  arc A232 (119.2151, -16.1083) -> (120.5264, -16.8366) centre (119.8708, -16.4725) ccw
  line L245 (119.2151, -16.1083) -> (120.0261, -14.6484)
  arc A233 (121.3374, -15.3767) -> (120.0261, -14.6484) centre (120.6817, -15.0125) ccw
  line L246 (126.9692, -13.9842) -> (126.9298, -14.5628)
  arc A234 (125.4333, -14.4608) -> (126.9298, -14.5628) centre (126.1815, -14.5118) ccw
  line L247 (125.4333, -14.4608) -> (125.4727, -13.8822)
  arc A235 (126.9692, -13.9842) -> (125.4727, -13.8822) centre (126.221, -13.9332) ccw
  line L248 (83.2374, -34.4267) -> (82.4264, -35.8866)
  arc A236 (81.1151, -35.1583) -> (82.4264, -35.8866) centre (81.7708, -35.5225) ccw
  line L249 (81.1151, -35.1583) -> (81.9261, -33.6984)
  arc A237 (83.2374, -34.4267) -> (81.9261, -33.6984) centre (82.5817, -34.0625) ccw
  line L250 (88.8692, -33.0342) -> (88.8298, -33.6128)
  arc A238 (87.3333, -33.5108) -> (88.8298, -33.6128) centre (88.0815, -33.5618) ccw
  line L251 (87.3333, -33.5108) -> (87.3727, -32.9322)
  arc A239 (88.8692, -33.0342) -> (87.3727, -32.9322) centre (88.121, -32.9832) ccw
  line L252 (111.8124, 41.7733) -> (111.0014, 40.3134)
  arc A240 (109.6902, 41.0417) -> (111.0014, 40.3134) centre (110.3458, 40.6775) ccw
  line L253 (109.6902, 41.0417) -> (110.5011, 42.5016)
  arc A241 (111.8124, 41.7733) -> (110.5011, 42.5016) centre (111.1567, 42.1375) ccw
  line L254 (117.4442, 43.1658) -> (117.4048, 42.5872)
  arc A242 (115.9083, 42.6892) -> (117.4048, 42.5872) centre (116.6565, 42.6382) ccw
  line L255 (115.9083, 42.6892) -> (115.9477, 43.2678)
  arc A243 (117.4442, 43.1658) -> (115.9477, 43.2678) centre (116.696, 43.2168) ccw
  line L256 (116.5749, 22.7233) -> (115.7639, 21.2634)
  arc A244 (114.4527, 21.9917) -> (115.7639, 21.2634) centre (115.1083, 21.6275) ccw
  line L257 (114.4527, 21.9917) -> (115.2636, 23.4516)
  arc A245 (116.5749, 22.7233) -> (115.2636, 23.4516) centre (115.9192, 23.0875) ccw
  line L258 (122.2067, 24.1158) -> (122.1673, 23.5372)
  arc A246 (120.6708, 23.6392) -> (122.1673, 23.5372) centre (121.419, 23.5882) ccw
  line L259 (120.6708, 23.6392) -> (120.7102, 24.2178)
  arc A247 (122.2067, 24.1158) -> (120.7102, 24.2178) centre (121.4585, 24.1668) ccw
  line L260 (140.3873, 3.6733) -> (139.5764, 2.2134)
  arc A248 (138.2652, 2.9417) -> (139.5764, 2.2134) centre (138.9208, 2.5775) ccw
  line L261 (138.2652, 2.9417) -> (139.0761, 4.4016)
  arc A249 (140.3873, 3.6733) -> (139.0761, 4.4016) centre (139.7317, 4.0375) ccw
  line L262 (146.0192, 5.0658) -> (145.9798, 4.4872)
  arc A250 (144.4833, 4.5892) -> (145.9798, 4.4872) centre (145.2315, 4.5382) ccw
  line L263 (144.4833, 4.5892) -> (144.5227, 5.1678)
  arc A251 (146.0192, 5.0658) -> (144.5227, 5.1678) centre (145.271, 5.1168) ccw
  line L264 (140.3873, -15.3767) -> (139.5764, -16.8366)
  arc A252 (138.2652, -16.1083) -> (139.5764, -16.8366) centre (138.9208, -16.4725) ccw
  line L265 (138.2652, -16.1083) -> (139.0761, -14.6484)
  arc A253 (140.3873, -15.3767) -> (139.0761, -14.6484) centre (139.7317, -15.0125) ccw
  line L266 (146.0192, -13.9842) -> (145.9798, -14.5628)
  arc A254 (144.4833, -14.4608) -> (145.9798, -14.5628) centre (145.2315, -14.5118) ccw
  line L267 (144.4833, -14.4608) -> (144.5227, -13.8822)
  arc A255 (146.0192, -13.9842) -> (144.5227, -13.8822) centre (145.271, -13.9332) ccw
  line L268 (121.3374, -34.4267) -> (120.5264, -35.8866)
  arc A256 (119.2151, -35.1583) -> (120.5264, -35.8866) centre (119.8708, -35.5225) ccw
  line L269 (119.2151, -35.1583) -> (120.0261, -33.6984)
  arc A257 (121.3374, -34.4267) -> (120.0261, -33.6984) centre (120.6817, -34.0625) ccw
  line L270 (126.9692, -33.0342) -> (126.9298, -33.6128)
  arc A258 (125.4333, -33.5108) -> (126.9298, -33.6128) centre (126.1815, -33.5618) ccw
  line L271 (125.4333, -33.5108) -> (125.4727, -32.9322)
  arc A259 (126.9692, -33.0342) -> (125.4727, -32.9322) centre (126.221, -32.9832) ccw
  line L272 (140.3873, 41.7733) -> (139.5764, 40.3134)
  arc A260 (138.2652, 41.0417) -> (139.5764, 40.3134) centre (138.9208, 40.6775) ccw
  line L273 (138.2652, 41.0417) -> (139.0761, 42.5016)
  arc A261 (140.3873, 41.7733) -> (139.0761, 42.5016) centre (139.7317, 42.1375) ccw
  line L274 (146.0192, 43.1658) -> (145.9798, 42.5872)
  arc A262 (144.4833, 42.6892) -> (145.9798, 42.5872) centre (145.2315, 42.6382) ccw
  line L275 (144.4833, 42.6892) -> (144.5227, 43.2678)
  arc A263 (146.0192, 43.1658) -> (144.5227, 43.2678) centre (145.271, 43.2168) ccw
  line L276 (140.3873, 22.7233) -> (139.5764, 21.2634)
  arc A264 (138.2652, 21.9917) -> (139.5764, 21.2634) centre (138.9208, 21.6275) ccw
  line L277 (138.2652, 21.9917) -> (139.0761, 23.4516)
  arc A265 (140.3873, 22.7233) -> (139.0761, 23.4516) centre (139.7317, 23.0875) ccw
  line L278 (146.0192, 24.1158) -> (145.9798, 23.5372)
  arc A266 (144.4833, 23.6392) -> (145.9798, 23.5372) centre (145.2315, 23.5882) ccw
  line L279 (144.4833, 23.6392) -> (144.5227, 24.2178)
  arc A267 (146.0192, 24.1158) -> (144.5227, 24.2178) centre (145.271, 24.1668) ccw
  line L280 (140.3873, -34.4267) -> (139.5764, -35.8866)
  arc A268 (138.2652, -35.1583) -> (139.5764, -35.8866) centre (138.9208, -35.5225) ccw
  line L281 (138.2652, -35.1583) -> (139.0761, -33.6984)
  arc A269 (140.3873, -34.4267) -> (139.0761, -33.6984) centre (139.7317, -34.0625) ccw
  line L282 (146.0192, -33.0342) -> (145.9798, -33.6128)
  arc A270 (144.4833, -33.5108) -> (145.9798, -33.6128) centre (145.2315, -33.5618) ccw
  line L283 (144.4833, -33.5108) -> (144.5227, -32.9322)
  arc A271 (146.0192, -33.0342) -> (144.5227, -32.9322) centre (145.271, -32.9832) ccw
  line L284 (102.2874, -34.4267) -> (101.4764, -35.8866)
  arc A272 (100.1651, -35.1583) -> (101.4764, -35.8866) centre (100.8208, -35.5225) ccw
  line L285 (100.1651, -35.1583) -> (100.9761, -33.6984)
  arc A273 (102.2874, -34.4267) -> (100.9761, -33.6984) centre (101.6317, -34.0625) ccw
  line L286 (107.9192, -33.0342) -> (107.8798, -33.6128)
  arc A274 (106.3833, -33.5108) -> (107.8798, -33.6128) centre (107.1315, -33.5618) ccw
  line L287 (106.3833, -33.5108) -> (106.4227, -32.9322)
  arc A275 (107.9192, -33.0342) -> (106.4227, -32.9322) centre (107.171, -32.9832) ccw
  line L288 (95.1436, -15.3767) -> (94.3327, -16.8366)
  arc A276 (93.0214, -16.1083) -> (94.3327, -16.8366) centre (93.677, -16.4725) ccw
  line L289 (93.0214, -16.1083) -> (93.8323, -14.6484)
  arc A277 (95.1436, -15.3767) -> (93.8323, -14.6484) centre (94.488, -15.0125) ccw
  line L290 (100.7755, -13.9842) -> (100.736, -14.5628)
  arc A278 (99.2395, -14.4608) -> (100.736, -14.5628) centre (99.9878, -14.5118) ccw
  line L291 (99.2395, -14.4608) -> (99.279, -13.8822)
  arc A279 (100.7755, -13.9842) -> (99.279, -13.8822) centre (100.0272, -13.9332) ccw
  circle A280 centre (-139.1188, 33.375) radius 0.35
  circle A281 centre (-146.9187, 33.375) radius 0.35
  circle A282 centre (-112.925, -42.825) radius 0.35
  circle A283 centre (-120.725, -42.825) radius 0.35
  circle A284 centre (-89.1125, -42.825) radius 0.35
  circle A285 centre (-96.9125, -42.825) radius 0.35
  circle A286 centre (-101.0187, 33.375) radius 0.35
  circle A287 centre (-108.8188, 33.375) radius 0.35
  circle A288 centre (-91.4938, 14.325) radius 0.35
  circle A289 centre (-99.2938, 14.325) radius 0.35
  circle A290 centre (-86.7313, -4.725) radius 0.35
  circle A291 centre (-94.5312, -4.725) radius 0.35
  circle A292 centre (-77.2062, -23.775) radius 0.35
  circle A293 centre (-85.0062, -23.775) radius 0.35
  circle A294 centre (-81.9688, 33.375) radius 0.35
  circle A295 centre (-89.7687, 33.375) radius 0.35
  circle A296 centre (-72.4437, 14.325) radius 0.35
  circle A297 centre (-80.2438, 14.325) radius 0.35
  circle A298 centre (-67.6813, -4.725) radius 0.35
  circle A299 centre (-75.4813, -4.725) radius 0.35
  circle A300 centre (-58.1563, -23.775) radius 0.35
  circle A301 centre (-65.9562, -23.775) radius 0.35
  circle A302 centre (-134.3562, 14.325) radius 0.35
  circle A303 centre (-142.1562, 14.325) radius 0.35
  circle A304 centre (-62.9188, 33.375) radius 0.35
  circle A305 centre (-70.7188, 33.375) radius 0.35
  circle A306 centre (-53.3938, 14.325) radius 0.35
  circle A307 centre (-61.1938, 14.325) radius 0.35
  circle A308 centre (-48.6313, -4.725) radius 0.35
  circle A309 centre (-56.4313, -4.725) radius 0.35
  circle A310 centre (-39.1063, -23.775) radius 0.35
  circle A311 centre (-46.9062, -23.775) radius 0.35
  circle A312 centre (-43.8687, 33.375) radius 0.35
  circle A313 centre (-51.6688, 33.375) radius 0.35
  circle A314 centre (-34.3438, 14.325) radius 0.35
  circle A315 centre (-42.1437, 14.325) radius 0.35
  circle A316 centre (-29.5813, -4.725) radius 0.35
  circle A317 centre (-37.3813, -4.725) radius 0.35
  circle A318 centre (-20.0562, -23.775) radius 0.35
  circle A319 centre (-27.8562, -23.775) radius 0.35
  circle A320 centre (-131.975, -4.725) radius 0.35
  circle A321 centre (-139.775, -4.725) radius 0.35
  circle A322 centre (-24.8188, 33.375) radius 0.35
  circle A323 centre (-32.6187, 33.375) radius 0.35
  circle A324 centre (-15.2937, 14.325) radius 0.35
  circle A325 centre (-23.0938, 14.325) radius 0.35
  circle A326 centre (-10.5312, -4.725) radius 0.35
  circle A327 centre (-18.3313, -4.725) radius 0.35
  circle A328 centre (-1.0063, -23.775) radius 0.35
  circle A329 centre (-8.8063, -23.775) radius 0.35
  circle A330 centre (-17.675, -42.825) radius 0.35
  circle A331 centre (-25.475, -42.825) radius 0.35
  circle A332 centre (-5.7688, 33.375) radius 0.35
  circle A333 centre (-13.5688, 33.375) radius 0.35
  circle A334 centre (3.7563, 14.325) radius 0.35
  circle A335 centre (-4.0438, 14.325) radius 0.35
  circle A336 centre (8.5188, -4.725) radius 0.35
  circle A337 centre (0.7188, -4.725) radius 0.35
  circle A338 centre (18.0437, -23.775) radius 0.35
  circle A339 centre (10.2438, -23.775) radius 0.35
  circle A340 centre (-127.2125, -23.775) radius 0.35
  circle A341 centre (-135.0125, -23.775) radius 0.35
  circle A342 centre (13.2812, 33.375) radius 0.35
  circle A343 centre (5.4813, 33.375) radius 0.35
  circle A344 centre (22.8063, 14.325) radius 0.35
  circle A345 centre (15.0063, 14.325) radius 0.35
  circle A346 centre (27.5688, -4.725) radius 0.35
  circle A347 centre (19.7688, -4.725) radius 0.35
  circle A348 centre (37.0938, -23.775) radius 0.35
  circle A349 centre (29.2938, -23.775) radius 0.35
  circle A350 centre (32.3312, 33.375) radius 0.35
  circle A351 centre (24.5312, 33.375) radius 0.35
  circle A352 centre (41.8563, 14.325) radius 0.35
  circle A353 centre (34.0562, 14.325) radius 0.35
  circle A354 centre (46.6188, -4.725) radius 0.35
  circle A355 centre (38.8188, -4.725) radius 0.35
  circle A356 centre (56.1437, -23.775) radius 0.35
  circle A357 centre (48.3438, -23.775) radius 0.35
  circle A358 centre (-136.7375, -42.825) radius 0.35
  circle A359 centre (-144.5375, -42.825) radius 0.35
  circle A360 centre (51.3813, 33.375) radius 0.35
  circle A361 centre (43.5813, 33.375) radius 0.35
  circle A362 centre (60.9062, 14.325) radius 0.35
  circle A363 centre (53.1063, 14.325) radius 0.35
  circle A364 centre (65.6688, -4.725) radius 0.35
  circle A365 centre (57.8688, -4.725) radius 0.35
  circle A366 centre (75.1937, -23.775) radius 0.35
  circle A367 centre (67.3937, -23.775) radius 0.35
  circle A368 centre (51.3813, -42.825) radius 0.35
  circle A369 centre (43.5813, -42.825) radius 0.35
  circle A370 centre (70.4313, 33.375) radius 0.35
  circle A371 centre (62.6313, 33.375) radius 0.35
  circle A372 centre (79.9563, 14.325) radius 0.35
  circle A373 centre (72.1562, 14.325) radius 0.35
  circle A374 centre (84.7188, -4.725) radius 0.35
  circle A375 centre (76.9188, -4.725) radius 0.35
  circle A376 centre (101.3875, -23.775) radius 0.35
  circle A377 centre (93.5875, -23.775) radius 0.35
  circle A378 centre (-120.0688, 33.375) radius 0.35
  circle A379 centre (-127.8688, 33.375) radius 0.35
  circle A380 centre (70.4313, -42.825) radius 0.35
  circle A381 centre (62.6313, -42.825) radius 0.35
  circle A382 centre (89.4813, 33.375) radius 0.35
  circle A383 centre (81.6813, 33.375) radius 0.35
  circle A384 centre (99.0062, 14.325) radius 0.35
  circle A385 centre (91.2063, 14.325) radius 0.35
  circle A386 centre (115.675, -4.725) radius 0.35
  circle A387 centre (107.875, -4.725) radius 0.35
  circle A388 centre (127.5813, -23.775) radius 0.35
  circle A389 centre (119.7812, -23.775) radius 0.35
  circle A390 centre (89.4813, -42.825) radius 0.35
  circle A391 centre (81.6813, -42.825) radius 0.35
  circle A392 centre (118.0563, 33.375) radius 0.35
  circle A393 centre (110.2562, 33.375) radius 0.35
  circle A394 centre (122.8187, 14.325) radius 0.35
  circle A395 centre (115.0187, 14.325) radius 0.35
  circle A396 centre (146.6313, -4.725) radius 0.35
  circle A397 centre (138.8313, -4.725) radius 0.35
  circle A398 centre (146.6313, -23.775) radius 0.35
  circle A399 centre (138.8313, -23.775) radius 0.35
  circle A400 centre (-110.5438, 14.325) radius 0.35
  circle A401 centre (-118.3438, 14.325) radius 0.35
  circle A402 centre (127.5813, -42.825) radius 0.35
  circle A403 centre (119.7812, -42.825) radius 0.35
  circle A404 centre (146.6313, 33.375) radius 0.35
  circle A405 centre (138.8313, 33.375) radius 0.35
  circle A406 centre (146.6313, 14.325) radius 0.35
  circle A407 centre (138.8313, 14.325) radius 0.35
  circle A408 centre (108.5312, -42.825) radius 0.35
  circle A409 centre (100.7313, -42.825) radius 0.35
  circle A410 centre (146.6313, -42.825) radius 0.35
  circle A411 centre (138.8313, -42.825) radius 0.35
  circle A412 centre (-105.7812, -4.725) radius 0.35
  circle A413 centre (-113.5813, -4.725) radius 0.35
  circle A414 centre (-96.2562, -23.775) radius 0.35
  circle A415 centre (-104.0563, -23.775) radius 0.35
  circle A416 centre (-148.375, 28) radius 1.1
  circle A417 centre (-104.875, -29) radius 1.1
  circle A418 centre (133.125, 28.5) radius 1.1
  circle A419 centre (114.125, -29) radius 1.1
  circle A420 centre (-4.875, 9) radius 1.1
  circle A421 centre (-143.0188, 38.1375) radius 1.994
  circle A422 centre (-148.0987, 38.1375) radius 0.851
  circle A423 centre (-137.9387, 38.1375) radius 0.851
  circle A424 centre (-116.825, -38.0625) radius 1.994
  circle A425 centre (-121.905, -38.0625) radius 0.851
  circle A426 centre (-111.745, -38.0625) radius 0.851
  circle A427 centre (-93.0125, -38.0625) radius 1.994
  circle A428 centre (-98.0925, -38.0625) radius 0.851
  circle A429 centre (-87.9325, -38.0625) radius 0.851
  circle A430 centre (-104.9188, 38.1375) radius 1.994
  circle A431 centre (-109.9988, 38.1375) radius 0.851
  circle A432 centre (-99.8388, 38.1375) radius 0.851
  circle A433 centre (-95.3937, 19.0875) radius 1.994
  circle A434 centre (-100.4738, 19.0875) radius 0.851
  circle A435 centre (-90.3137, 19.0875) radius 0.851
  circle A436 centre (-90.6312, 0.0375) radius 1.994
  circle A437 centre (-95.7113, 0.0375) radius 0.851
  circle A438 centre (-85.5513, 0.0375) radius 0.851
  circle A439 centre (-81.1063, -19.0125) radius 1.994
  circle A440 centre (-86.1863, -19.0125) radius 0.851
  circle A441 centre (-76.0263, -19.0125) radius 0.851
  circle A442 centre (-85.8688, 38.1375) radius 1.994
  circle A443 centre (-90.9488, 38.1375) radius 0.851
  circle A444 centre (-80.7887, 38.1375) radius 0.851
  circle A445 centre (-76.3438, 19.0875) radius 1.994
  circle A446 centre (-81.4237, 19.0875) radius 0.851
  circle A447 centre (-71.2638, 19.0875) radius 0.851
  circle A448 centre (-71.5812, 0.0375) radius 1.994
  circle A449 centre (-76.6612, 0.0375) radius 0.851
  circle A450 centre (-66.5012, 0.0375) radius 0.851
  circle A451 centre (-62.0563, -19.0125) radius 1.994
  circle A452 centre (-67.1363, -19.0125) radius 0.851
  circle A453 centre (-56.9763, -19.0125) radius 0.851
  circle A454 centre (-138.2562, 19.0875) radius 1.994
  circle A455 centre (-143.3363, 19.0875) radius 0.851
  circle A456 centre (-133.1763, 19.0875) radius 0.851
  circle A457 centre (-66.8187, 38.1375) radius 1.994
  circle A458 centre (-71.8988, 38.1375) radius 0.851
  circle A459 centre (-61.7388, 38.1375) radius 0.851
  circle A460 centre (-57.2938, 19.0875) radius 1.994
  circle A461 centre (-62.3738, 19.0875) radius 0.851
  circle A462 centre (-52.2138, 19.0875) radius 0.851
  circle A463 centre (-52.5313, 0.0375) radius 1.994
  circle A464 centre (-57.6112, 0.0375) radius 0.851
  circle A465 centre (-47.4513, 0.0375) radius 0.851
  circle A466 centre (-43.0063, -19.0125) radius 1.994
  circle A467 centre (-48.0862, -19.0125) radius 0.851
  circle A468 centre (-37.9263, -19.0125) radius 0.851
  circle A469 centre (-47.7687, 38.1375) radius 1.994
  circle A470 centre (-52.8488, 38.1375) radius 0.851